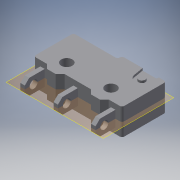
# Autodesk Inventor part: body
Saved by Autodesk Inventor 2018 (Build 220112000, 112)
## iProperties
Created: 2017-11-12
Part Number: body
Material: Generic
Document SubType Name: Modeling
Designer: leo2a
Density: 1 g/cm^3
Appearance: Default
Author: leo2a
Autodesk Inventor part; units mm, degrees
ref_plane "YZ Plane" through (0, 0, 0) normal (1, 0, 0) x (0, 1, 0)
ref_plane "XZ Plane" through (0, 0, 0) normal (0, 1, 0) x (-1, 0, 0)
ref_plane "XY Plane" through (0, 0, 0) normal (0, 0, 1) x (1, 0, 0)
sketch "Sketch1" plane through (0, 0, 0) normal (0, 0, 1) x (1, 0, 0)
  line L0 (-10, -5) -> (10, -5)
  line L1 (10, -5) -> (10, 5)
  line L2 (10, 5) -> (-10, 5)
  line L3 (-10, 5) -> (-10, -5)
  line L4 (-10, -5) -> (10, 5) construction
  line L5 (10, -5) -> (-10, 5) construction
  point P0 (0, 0)
  dimension "d0" = 20
  dimension "d1" = 10
  constraints: 12 end point, 2 midpoint, 2 parallel, 1 horizontal, 1 perpendicular
  measures "d0" distance of L0.start L0.end
  measures "d1" distance of L1.end L0.end
extrude "Extrusion1" add sketch "Sketch1" along normal blind 6
sketch "Sketch2" plane through (-10, 5, 0) normal (0, 1, 0) x (1, 0, 0)
  line L0 (0, -6) -> (20, -6) projected
  line L1 (0, 0) -> (10, 0)
  line L2 (10, 0) -> (10, -6)
  line L3 (10, -6) -> (0, -6)
  line L4 (0, -6) -> (0, 0)
  constraints: 8 end point, 2 parallel, 1 horizontal, 1 midpoint, 1 perpendicular
extrude "Extrusion2" cut sketch "Sketch2" against normal blind 1
sketch "Sketch3" plane through (0, 0, 6) normal (0, 0, 1) x (1, 0, 0)
  line L0 (-10, -5) -> (10, -5) projected
  line L1 (-10, -5) -> (-10, -2.5)
  line L2 (-10, 4) -> (-10, -5) projected
  line L3 (-10, -2.5) -> (-5, -2.5)
  circle A0 centre (-5, -2.5) radius 1.25
  line L4 (10, -5) -> (5, -5)
  line L5 (5, -5) -> (5, -2.5)
  circle A1 centre (5, -2.5) radius 1.25
  point P0 (0, 0)
  dimension "d6" = 2.5
  dimension "d7" = 5
  dimension "d8" = 2.5
  dimension "d9" = 5
  dimension "d10" = 2.5
  constraints: 8 end point, 2 centre point, 2 coincident, 2 perpendicular, 2 point on line
  measures "d6" distance of L0.start L1.end
  measures "d7" distance of L1.end L3.end
  measures "d8" diameter of A0
  measures "d9" distance of L0.end L4.end
  measures "d10" diameter of A1
extrude "Extrusion3" cut sketch "Sketch3" against normal through all
sketch "Sketch4" plane through (-10, -5, 0) normal (0, -1, 0) x (1, 0, 0)
  line L0 (20, 0) -> (20, 6) projected
  line L1 (20, 3) -> (18, 3)
  line L2 (18.5, 4.75) -> (18.5, 1.25)
  line L3 (18.5, 1.25) -> (17.5, 1.25)
  line L4 (17.5, 1.25) -> (17.5, 4.75)
  line L5 (17.5, 4.75) -> (18.5, 4.75)
  line L6 (18.5, 4.75) -> (17.5, 1.25) construction
  line L7 (18.5, 1.25) -> (17.5, 4.75) construction
  line L8 (0, 0) -> (0, 6) projected
  line L9 (0, 3) -> (2, 3)
  line L10 (2.5002, 1.25) -> (2.5002, 4.75)
  line L11 (2.5002, 4.75) -> (1.4998, 4.75)
  line L12 (1.4998, 4.75) -> (1.4998, 1.25)
  line L13 (1.4998, 1.25) -> (2.5002, 1.25)
  line L14 (2.5002, 1.25) -> (1.4998, 4.75) construction
  line L15 (2.5002, 4.75) -> (1.4998, 1.25) construction
  line L16 (2, 3) -> (9.5, 3)
  line L17 (10, 1.25) -> (10, 4.75)
  line L18 (10, 4.75) -> (9, 4.75)
  line L19 (9, 4.75) -> (9, 1.25)
  line L20 (9, 1.25) -> (10, 1.25)
  line L21 (10, 1.25) -> (9, 4.75) construction
  line L22 (10, 4.75) -> (9, 1.25) construction
  point P0 (10, 0)
  dimension "d13" = 2
  dimension "d14" = 3.5
  dimension "d15" = 1
  dimension "d16" = 2
  dimension "d17" = 7.5
  dimension "d18" = 1
  constraints: 42 end point, 8 midpoint, 6 parallel, 4 perpendicular, 3 horizontal, 2 vertical
  measures "d13" distance of L1.start L1.end
  measures "d14" distance of L2.start L2.end
  measures "d15" distance of L2.end L3.end
  measures "d16" distance of L9.start L9.end
  measures "d17" distance of L9.end L16.end
  measures "d18" distance of L18.end L17.end
extrude "Extrusion4" add sketch "Sketch4" along normal blind 4.5
chamfer "Chamfer1" distance 1 angle 45 6 edges at (8, -9.5, 4.75) (8, -9.5, 1.25) (-0.5, -9.5, 1.25) (-0.5, -9.5, 4.75) (-8, -9.5, 1.25) (-8, -9.5, 4.75)
sketch "Sketch5" plane through (8.5, -5, 4.75) normal (1, 0, 0) x (0, 0, -1)
  line L0 (1, -4.5) -> (2.5, -4.5) projected
  line L1 (1.75, -4.5) -> (1.75, -2.5)
  circle A0 centre (1.75, -2.5) radius 0.9
  point P0 (4.75, 5)
  dimension "d24" = 2
  dimension "d25" = 1.8
  constraints: 2 end point, 1 centre point, 1 coincident, 1 midpoint, 1 vertical
  measures "d24" distance of L1.start L1.end
  measures "d25" diameter of A0
extrude "Extrusion5" cut sketch "Sketch5" against normal up to surface (17.0002 mm away)
sketch "Sketch6" plane through (-10, -5, 0) normal (0, -1, 0) x (1, 0, 0)
  line L0 (0, 6) -> (20, 6) projected
  line L1 (0, 6) -> (3, 6)
  line L2 (3, 6) -> (3, 0)
  line L3 (0, 0) -> (20, 0) projected
  line L4 (3, 0) -> (8, 0)
  line L5 (8, 6) -> (3, 6)
  line L6 (3, 6) -> (7, 6)
  line L7 (7, 6) -> (7, 0)
  point P0 (10, 0)
  dimension "d28" = 3
  dimension "d29" = 5
  dimension "d42" = 4
  constraints: 12 end point, 5 point on line, 3 perpendicular
  measures "d28" distance of L0.start L1.end
  measures "d29" distance of L2.end L4.end
  measures "d42" distance of L1.end L6.end
extrude "Extrusion6" add sketch "Sketch6" along normal blind 1
chamfer "Chamfer2" distance 1 angle 45 2 edges at (-7, -6, 3) (-3, -6, 3)
sketch "Sketch7" plane through (10, -5, 0) normal (0, -1, 0) x (1, 0, 0)
  line L0 (0, 0) -> (-3, 0)
  line L1 (-3, 0) -> (-3, 6)
  line L2 (0, 6) -> (-10, 6) projected
  line L3 (-3, 6) -> (-7, 6)
  line L4 (-6.25, 6) -> (-3.75, 6) projected
  line L5 (-7, 6) -> (-7, 0)
  line L6 (0, 0) -> (-10, 0) projected
  line L7 (-3, 0) -> (-7, 0)
  dimension "d35" = 3
  dimension "d36" = 4
  constraints: 10 end point, 2 collinear, 2 perpendicular, 2 point on line, 1 horizontal
  measures "d35" distance of L0.start L0.end
  measures "d36" distance of L1.end L3.end
extrude "Extrusion7" add sketch "Sketch7" along normal blind 1
chamfer "Chamfer3" distance 1 angle 45 2 edges at (7, -6, 3) (3, -6, 3)
sketch "Sketch8" plane through (0, 0, 6) normal (0, 0, 1) x (1, 0, 0)
  line L0 (8, 5) -> (5, 5)
  arc A0 (5, 3) -> (8, 3) centre (6.5, 3) ccw
  line L1 (5, 3) -> (4.6473, 5)
  line L2 (10, 5) -> (0, 5) projected
  line L3 (5, 3) -> (7.0309, 3) construction
  line L4 (8, 3) -> (8.3527, 5)
  line L5 (8, 3) -> (10.0309, 3) construction
  line L6 (8.3527, 5) -> (8, 5)
  line L7 (5, 5) -> (4.6473, 5)
  point P0 (0, 0)
  dimension "d52" = 100
  dimension "d53" = 80
  constraints: 14 end point, 2 collinear, 2 equal length, 2 horizontal, 2 point on circle, 2 point on line, 1 centre point
  measures "d52" angle of L3 L1
  measures "d53" angle of L5 L4
extrude "Extrusion8" cut sketch "Sketch8" against normal blind 0.5
ref_plane "Work Plane1" through (0, 0, 3) normal (0, 0, 1) x (1, 0, 0)
sketch "Sketch10" plane through (0, 0, 5.5) normal (0, 0, 1) x (1, 0, 0)
  arc A0 (5, 3) -> (8, 3) centre (6.5, 3) ccw projected
  circle A1 centre (6.5, 3) radius 0.75
  point P0 (0, 0)
  dimension "d48" = 1.5
  constraints: 1 centre point, 1 coincident
  measures "d48" diameter of A1
extrude "Extrusion9" add sketch "Sketch10" along normal blind 0.5
mirror "Mirror1" about plane through (0, 0, 3) normal (0, 0, 1) of "Extrusion9", "Extrusion8"
fillet "Fillet1" radius 0.5 6 edges at (-10, 4, 3) (0, 5, 3) (0, 4, 3) (10, 5, 3) (10, -5, 3) (-10, -5, 3)
body "Solid1"
